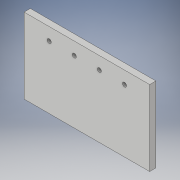
# Autodesk Inventor part: Extender_pulley_gusset
Saved by Autodesk Inventor 2018 (Build 220112000, 112)
## iProperties
Created: 2018-08-30
Part Number: Extender_pulley_gusset
Material: Generic
Document SubType Name: Modeling
Designer: baoan
Density: 1 g/cm^3
Appearance: Default
Author: baoan
Autodesk Inventor part; units mm, degrees
ref_plane "YZ Plane" through (0, 0, 0) normal (1, 0, 0) x (0, 1, 0)
ref_plane "XZ Plane" through (0, 0, 0) normal (0, 1, 0) x (-1, 0, 0)
ref_plane "XY Plane" through (0, 0, 0) normal (0, 0, 1) x (1, 0, 0)
sketch "Sketch1" plane through (0, 0, 0) normal (0, 0, 1) x (1, 0, 0)
  line L0 (-63.5, -38.1) -> (63.5, -38.1)
  line L1 (63.5, -38.1) -> (63.5, 38.1)
  line L2 (63.5, 38.1) -> (-63.5, 38.1)
  line L3 (-63.5, 38.1) -> (-63.5, -38.1)
  line L4 (-63.5, -38.1) -> (63.5, 38.1) construction
  line L5 (63.5, -38.1) -> (-63.5, 38.1) construction
  point P0 (0, 0)
  dimension "d0" = 127
  dimension "d1" = 76.2
  constraints: 12 end point, 2 midpoint, 2 parallel, 1 horizontal, 1 perpendicular
  measures "d0" distance of L2.end L1.end
  measures "d1" distance of L1.end L0.end
extrude "Extrusion1" add sketch "Sketch1" along normal mid plane 6.35
sketch "Sketch2" plane through (0, 0, 3.175) normal (0, 0, 1) x (1, 0, 0)
  line L0 (-63.5, 38.1) -> (-63.5, -38.1) projected
  line L1 (63.5, 38.1) -> (-63.5, 38.1) projected
  point P0 (0, 0)
  point P1 (-38.1, 25.4)
  point P2 (-12.7, 25.4)
  point P3 (12.7, 25.4)
  point P4 (38.1, 25.4)
  dimension "d4" = 25.4
  dimension "d5" = 25.4
  dimension "d6" = 25.4
  dimension "d8" = 25.4
  dimension "d9" = 12.7
  constraints: 3 horizontal alignment
  measures "d4" distance of point (-12.7, 25.4) point (-38.1, 25.4)
  measures "d5" distance of point (12.7, 25.4) point (-12.7, 25.4)
  measures "d6" distance of point (38.1, 25.4) point (12.7, 25.4)
  measures "d8" distance from line of L0 point (-38.1, 25.4)
  measures "d9" distance from line of L1 point (-38.1, 25.4)
hole "Hole1" at (-38.1, 25.4, 3.175) at (-12.7, 25.4, 3.175) at (12.7, 25.4, 3.175) at (38.1, 25.4, 3.175) direction (0, 0, -1) diameter 4.1402 end through all
body "Solid1"
